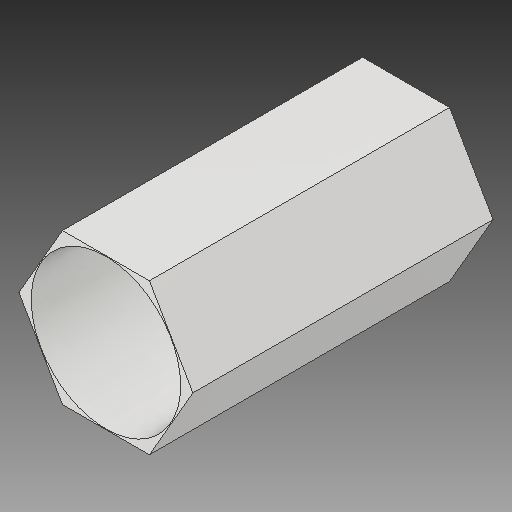
# Autodesk Inventor part: 2AM-17-P-1202 - hex to tube adapter
Saved by Autodesk Inventor 2017 (Build 210142000, 142)
## iProperties
Created: 2017-12-27
Part Number: 2AM-17-P-1202 - hex to tube adapter
Material: ABS Plastic
Document SubType Name: Modeling
Designer: Micah
Density: 1.06 g/cm^3
Appearance: Smooth - White
Author: Micah
Autodesk Inventor part; units mm, degrees
ref_plane "YZ Plane" through (0, 0, 0) normal (1, 0, 0) x (0, 1, 0)
ref_plane "XZ Plane" through (0, 0, 0) normal (0, 1, 0) x (-1, 0, 0)
ref_plane "XY Plane" through (0, 0, 0) normal (0, 0, 1) x (1, 0, 0)
sketch "Sketch1" plane through (0, 0, 0) normal (0, 0, 1) x (1, 0, 0)
  line L0 (-3.6808, 6.3754) -> (3.6808, 6.3754)
  line L1 (3.6808, 6.3754) -> (7.3617, 0)
  line L2 (3.6808, -6.3754) -> (-3.6808, -6.3754)
  line L3 (-3.6808, -6.3754) -> (-7.3617, 0)
  line L4 (-3.6808, 6.3754) -> (-7.3617, 0)
  line L5 (3.6808, -6.3754) -> (7.3617, 0)
  circle A0 centre (0, 0) radius 6.3246
  dimension "d0" = 12.6492
  constraints: 12 end point, 1 centre point, 1 coincident, 1 horizontal, 1 parallel
  measures "d0" diameter of A0
extrude "Extrusion1" add sketch "Sketch1" along normal blind 25.4
body "Solid1"
